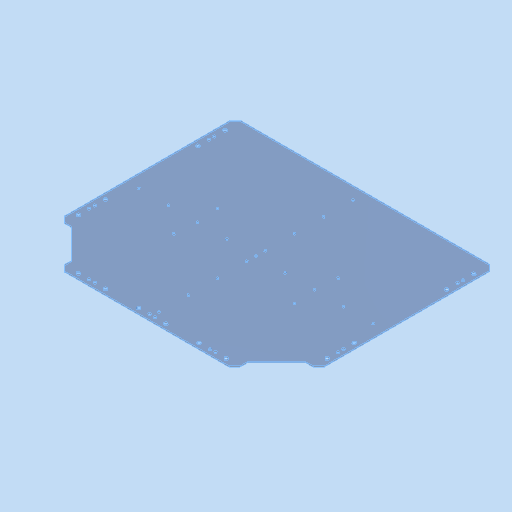
# Autodesk Inventor part: enc-FrontPanel Unten
Saved by Autodesk Inventor 2023.2 (Build 272271000, 271)
## iProperties
Created: 2023-11-30
Part Number: enc-FrontPanel Unten
Material: Generisch
Document SubType Name: Modeling
Designer: Nils Bade
Density: 1 g/cm^3
Appearance: PVC Verglasung
Description: Fertigung
Auf Bestellliste: True
Author: Nils Bade
Autodesk Inventor part; units mm, degrees
ref_plane "YZ Plane" through (0, 0, 0) normal (1, 0, 0) x (0, 1, 0)
ref_plane "XZ Plane" through (0, 0, 0) normal (0, 1, 0) x (-1, 0, 0)
ref_plane "XY Plane" through (0, 0, 0) normal (0, 0, 1) x (1, 0, 0)
sketch "Skizze1" plane through (0, 0, 0) normal (0, 1, 0) x (-1, 0, 0)
  line L0 (0, 0) -> (-710, 0)
  line L1 (-710, 0) -> (-710, 597)
  line L2 (-710, 597) -> (0, 597)
  line L3 (0, 597) -> (0, 0)
  line L4 (-355, 0) -> (-355, 597) construction
  line L5 (0, 298.5) -> (-710, 298.5) construction
  line L6 (-190, 0) -> (-190, 597) construction
  line L7 (-520, 0) -> (-520, 597) construction
  line L8 (-710, 407) -> (0, 407) construction
  line L9 (0, 80) -> (-710, 80) construction
  line L10 (-695, 582) -> (-695, 15) construction
  line L11 (-695, 15) -> (-15, 15) construction
  line L12 (-15, 15) -> (-15, 582) construction
  line L13 (-15, 582) -> (-695, 582) construction
  line L14 (-23, 362) -> (-7, 362) construction
  line L15 (-7, 362) -> (-7, 452) construction
  line L16 (-7, 452) -> (-23, 452) construction
  line L17 (-23, 452) -> (-23, 362) construction
  line L18 (-23, 362) -> (-7, 452) construction
  line L19 (-7, 362) -> (-23, 452) construction
  line L20 (-142.5, 590) -> (-237.5, 590) construction
  line L21 (-237.5, 590) -> (-237.5, 574) construction
  line L22 (-237.5, 574) -> (-142.5, 574) construction
  line L23 (-142.5, 574) -> (-142.5, 590) construction
  line L24 (-142.5, 590) -> (-237.5, 574) construction
  line L25 (-237.5, 590) -> (-142.5, 574) construction
  line L26 (-307.5, 590) -> (-402.5, 590) construction
  line L27 (-402.5, 590) -> (-402.5, 574) construction
  line L28 (-402.5, 574) -> (-307.5, 574) construction
  line L29 (-307.5, 574) -> (-307.5, 590) construction
  line L30 (-307.5, 590) -> (-402.5, 574) construction
  line L31 (-402.5, 590) -> (-307.5, 574) construction
  circle A0 centre (-15, 399.5) radius 3.25
  circle A1 centre (-15, 370) radius 4.5
  circle A2 centre (-15, 414.5) radius 3.25
  circle A3 centre (-15, 444) radius 4.5
  circle A4 centre (-182.5, 582) radius 3.25
  circle A5 centre (-153, 582) radius 4.5
  circle A6 centre (-318, 582) radius 4.5
  circle A7 centre (-347.5, 582) radius 3.25
  circle A8 centre (-197.5, 582) radius 3.25
  circle A9 centre (-227, 582) radius 4.5
  circle A10 centre (-392, 582) radius 4.5
  circle A11 centre (-362.5, 582) radius 3.25
  circle A12 centre (-695, 399.5) radius 3.25
  circle A13 centre (-695, 370) radius 4.5
  circle A14 centre (-695, 444) radius 4.5
  circle A15 centre (-695, 414.5) radius 3.25
  circle A16 centre (-527.5, 582) radius 3.25
  circle A17 centre (-557, 582) radius 4.5
  circle A18 centre (-512.5, 582) radius 3.25
  circle A19 centre (-483, 582) radius 4.5
  circle A20 centre (-15, 43) radius 4.5
  circle A21 centre (-15, 72.5) radius 3.25
  circle A22 centre (-190, 238.5) radius 2.75
  circle A23 centre (-190, 358.5) radius 2.75
  circle A24 centre (-520, 238.5) radius 2.75
  circle A25 centre (-520, 358.5) radius 2.75
  circle A26 centre (-15, 117) radius 4.5
  circle A27 centre (-15, 87.5) radius 3.25
  circle A28 centre (-695, 43) radius 4.5
  circle A29 centre (-695, 72.5) radius 3.25
  circle A30 centre (-695, 87.5) radius 3.25
  circle A31 centre (-695, 117) radius 4.5
  line L32 (-115, 597) -> (-115, 562)
  line L33 (-115, 562) -> (-35, 482)
  line L34 (-35, 482) -> (0, 482)
  line L35 (-595, 597) -> (-595, 562)
  line L36 (-595, 562) -> (-675, 482)
  line L37 (-675, 482) -> (-710, 482)
  point P0 (-15, 407)
  point P1 (-190, 582)
  point P2 (-355, 582)
  point P3 (-190, 298.5)
  dimension "d0" = 710
  dimension "d1" = 597
  dimension "d2" = 190
  dimension "d3" = 80
  dimension "d4" = 190
  dimension "d5" = 190
  dimension "d6" = 15
  dimension "d7" = 16
  dimension "d8" = 90
  dimension "d9" = 95
  dimension "d10" = 16
  dimension "d11" = 95
  dimension "d12" = 16
  dimension "d13" = 6.5
  dimension "d14" = 7.5
  dimension "d15" = 9
  dimension "d16" = 37
  dimension "d17" = 6.5
  dimension "d18" = 9
  dimension "d19" = 7.5
  dimension "d20" = 37
  dimension "d21" = 6.5
  dimension "d22" = 9
  dimension "d23" = 7.5
  dimension "d24" = 37
  dimension "d30" = 5.5
  dimension "d31" = 60
  dimension "d34" = 6.5
  dimension "d35" = 9
  dimension "d36" = 7.5
  dimension "d37" = 37
  dimension "d80" = 680
  dimension "d81" = 45
  dimension "d83" = 115
  dimension "d84" = 115
  dimension "d85" = 35
  constraints: 76 end point, 32 centre point, 27 symmetric about line, 23 point on line, 12 midpoint, 10 parallel, 10 perpendicular, 4 horizontal, 1 vertical, 26 other
  measures "d0" distance of L0.start L0.end
  measures "d1" distance of L2.end L0.start
  measures "d2" distance between parallel lines of L2 L8
  measures "d3" distance between parallel lines of L0 L9
  measures "d4" distance between parallel lines of L3 L6
  measures "d5" distance between parallel lines of L1 L7
  measures "d6" distance between parallel lines of L1 L10
  measures "d7" distance of L16.end L15.end
  measures "d8" distance of L15.end L14.end
  measures "d9" distance of L22.end L21.end
  measures "d10" distance of L21.end L20.end
  measures "d11" distance of L28.end L27.end
  measures "d12" distance of L27.end L26.end
  measures "d13" diameter of A0
  measures "d14" distance from line of L8 A0.centre
  measures "d15" diameter of A1
  measures "d16" distance from line of L8 A1.centre
  measures "d17" diameter of A4
  measures "d18" diameter of A5
  measures "d19" distance from line of L6 A4.centre
  measures "d20" distance from line of L6 A5.centre
  measures "d21" diameter of A7
  measures "d22" diameter of A6
  measures "d23" distance from line of L4 A7.centre
  measures "d24" distance from line of L4 A6.centre
  measures "d30" diameter of A22
  measures "d31" distance from line of L5 A22.centre
  measures "d34" diameter of A21
  measures "d35" diameter of A20
  measures "d36" distance from line of L9 A21.centre
  measures "d37" distance from line of L9 A20.centre
  measures "d80" distance between parallel lines of L10 L12
  measures "d81" angle of L2 L33
  measures "d83" distance between parallel lines of L3 L32
  measures "d84" distance between parallel lines of L2 L34
  measures "d85" distance of L32.start L32.end
extrude "Ex-Platte" add sketch "Skizze1" along normal blind 3 contours L0 L1 L37 L36 L35 L2 L32 L33 L34 L3
chamfer "Fase-15mm" distance 15 angle 45 6 edges at (710, 1.5, 0) (0, 1.5, 0) (0, 1.5, 482) (115, 1.5, 597) (595, 1.5, 597) (710, 1.5, 482)
sketch "Profil-Verstärkung" plane through (0, 0, 0) normal (0, 1, 0) x (-1, 0, 0)
  line L0 (-695, 0) -> (-15, 0) projected
  line L1 (0, 15) -> (0, 482) projected
  line L2 (-115, 597) -> (-595, 597) projected
  line L3 (-710, 482) -> (-710, 15) projected
  line L4 (0, 298.5) -> (-710, 298.5) construction
  circle A0 centre (-15, 117) radius 4.5 projected
  circle A1 centre (-15, 370) radius 4.5 projected
  circle A2 centre (-190, 358.5) radius 2.75 projected
  circle A3 centre (-190, 238.5) radius 2.75 projected
  circle A4 centre (-227, 582) radius 4.5 projected
  circle A5 centre (-318, 582) radius 4.5 projected
  line L5 (-355, 0) -> (-355, 597) construction
  circle A6 centre (-355, 298.5) radius 2.5
  circle A7 centre (-435, 298.5) radius 2.5
  circle A8 centre (-515, 298.5) radius 2.5
  circle A9 centre (-595, 298.5) radius 2.5
  circle A10 centre (-675, 298.5) radius 2.5
  circle A11 centre (-355, 323.5) radius 2.5
  circle A12 centre (-355, 403.5) radius 2.5
  circle A13 centre (-355, 483.5) radius 2.5
  circle A14 centre (-355, 563.5) radius 2.5
  circle A15 centre (-275, 298.5) radius 2.5
  circle A16 centre (-195, 298.5) radius 2.5
  circle A17 centre (-115, 298.5) radius 2.5
  circle A18 centre (-35, 298.5) radius 2.5
  circle A19 centre (-355, 273.5) radius 2.5
  circle A20 centre (-355, 193.5) radius 2.5
  circle A21 centre (-355, 113.5) radius 2.5
  circle A22 centre (-355, 33.5) radius 2.5
  point P0 (0, 0)
  point P1 (0, 582)
  point P2 (-15, 597)
  point P3 (-695, 597)
  point P4 (-710, 582)
  dimension "d38" = 710
  dimension "d40" = 121.5
  dimension "d42" = 11.5
  dimension "d61" = 5
  dimension "d64" = 80
  dimension "d69" = 5
  dimension "d70" = 25
  dimension "d73" = 80
  constraints: 17 centre point, 8 symmetric about line, 4 end point, 3 midpoint, 3 point on line, 1 horizontal, 1 vertical, 22 other
  measures "d38" distance of L4.start L4.end
  measures "d40" vertical distance of A0.centre A3.centre
  measures "d42" vertical distance of A1.centre A2.centre
  measures "d61" diameter of A6
  measures "d64" distance of A6.centre A7.centre
  measures "d69" diameter of A11
  measures "d70" distance of A6.centre A11.centre
  measures "d73" distance of A11.centre A12.centre
extrude "Ex-ProfilBohrungen" cut sketch "Profil-Verstärkung" along normal up to surface (3 mm away) contours A6 | A7 | A8 | A9 | A10 | A11 | A12 | A13 | A14 | A15 | A16 | A17 | A18 | A19 | A20 | A21 | A22
equation "\"d5\" = d4"
equation "\"d17\" = d13"
equation "\"d18\" = d15"
equation "\"d19\" = d14"
equation "\"d20\" = d16"
equation "\"d21\" = d13"
equation "\"d22\" = d15"
equation "\"d23\" = d14"
equation "\"d24\" = d16"
equation "\"d34\" = d13"
equation "\"d35\" = d15"
equation "\"d36\" = d14"
equation "\"d37\" = d16"
equation "\"d84\" = d83"
equation "\"d69\" = d61"
